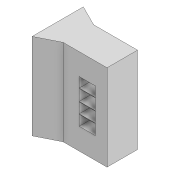
# Autodesk Inventor part: Sliding test insert
Saved by Autodesk Inventor 2020 (Build 240168000, 168)
## iProperties
Created: 2019-11-10
Part Number: Sliding test insert
Material: Generic
Document SubType Name: Modeling
Designer: ball
Density: 1 g/cm^3
Appearance: Default
Author: ball
Autodesk Inventor part; units mm, degrees
ref_plane "YZ Plane" through (0, 0, 0) normal (1, 0, 0) x (0, 1, 0)
ref_plane "XZ Plane" through (0, 0, 0) normal (0, 1, 0) x (-1, 0, 0)
ref_plane "XY Plane" through (0, 0, 0) normal (0, 0, 1) x (1, 0, 0)
sketch "Sketch1" plane through (0, 0, 0) normal (0, 1, 0) x (-1, 0, 0)
  line L0 (0, 4.5) -> (-12.7, 4.5)
  line L1 (-12.7, 4.5) -> (-12.7, -4.5)
  line L2 (-12.7, -4.5) -> (0, -4.5)
  line L3 (0, 4.5) -> (0.254, 4.5)
  line L4 (0.254, -4.5) -> (0, -4.5)
  line L5 (6.35, 4.5) -> (6.35, -4.5)
  line L6 (6.35, 7.548) -> (6.35, 4.5)
  line L7 (6.35, -7.548) -> (6.35, -4.5)
  line L8 (0.254, 4.5) -> (6.35, 7.548)
  line L9 (0.254, -4.5) -> (6.35, -7.548)
  point P0 (0, 0)
  point P1 (0, -4.5)
  dimension "d1" = 9
  dimension "d2" = 4.5
  dimension "d7" = 3.048
  dimension "d8" = 3.048
  dimension "d9" = 12.954
  dimension "d16" = 6.096
  constraints: 20 end point, 2 horizontal, 2 parallel, 2 point on line, 1 perpendicular
  measures "d1" distance of L1.end L0.end
  measures "d2" distance from line of L0 point (0, 0)
  measures "d7" distance from line of L6.start L0
  measures "d8" distance from line of L7.start L2
  measures "d9" distance from line of L4.start L1
  measures "d16" distance from line of L7 L4.start
extrude "Shape" add sketch "Sketch1" along normal blind 25.4
sketch "Sketch2" plane through (-0.254, 0, 4.5) normal (0, 0, 1) x (1, 0, 0)
  line L0 (4.7625, 19.05) -> (9.5125, 19.05)
  line L1 (9.5125, 19.05) -> (9.5125, 6.35)
  line L2 (9.5125, 6.35) -> (4.7625, 6.35)
  line L3 (4.7625, 6.35) -> (4.7625, 19.05)
  point P0 (0.254, 0)
  dimension "d12" = 4.75
  dimension "d13" = 12.7
  constraints: 8 end point, 2 parallel, 1 horizontal, 1 perpendicular
  measures "d12" distance of L1.end L2.end
  measures "d13" distance of L0.end L1.end
extrude "Bridge" cut sketch "Sketch2" against normal through all
sketch "Sketch3" plane through (4.5085, 6.35, 4.5) normal (1, 0, 0) x (0, 0, -1)
  line L0 (9, 12.7) -> (9, 0) construction
  line L1 (0, 12.7) -> (9, 12.7) construction
  line L2 (9, 0) -> (0, 0) construction
  line L3 (0, -6.35) -> (0, 19.05) projected
  line L4 (9, -6.35) -> (9, 19.05) projected
  line L5 (0, 9.7549) -> (9, 9.7549)
  line L6 (9, 9.7549) -> (9, 9.6279)
  line L7 (9, 9.6279) -> (0, 9.6279)
  line L8 (0, 9.6279) -> (0, 9.7549)
  line L9 (0, 6.35) -> (9, 6.35)
  line L10 (9, 6.35) -> (9, 6.223)
  line L11 (9, 6.223) -> (0, 6.223)
  line L12 (0, 6.223) -> (0, 6.35)
  line L13 (0, 3.175) -> (9, 3.175)
  line L14 (9, 3.175) -> (9, 3.048)
  line L15 (9, 3.048) -> (0, 3.048)
  line L16 (0, 3.048) -> (0, 3.175)
  point P0 (4.5, -6.35)
  point P1 (0, 3.048)
  point P2 (0, 6.223)
  point P3 (9, 6.35)
  point P4 (0, 9.6279)
  point P5 (9, 9.7549)
  dimension "d17" = 0.127
  dimension "d18" = 0.127
  dimension "d19" = 0.127
  dimension "d20" = 2.9451
  dimension "d22" = 9.525
  constraints: 28 end point, 6 parallel, 5 horizontal, 4 point on line, 3 perpendicular, 1 midpoint
  measures "d17" distance of L5.end L6.end
  measures "d18" distance of L9.end L10.end
  measures "d19" distance of L13.end L14.end
  measures "d20" distance between parallel lines of L1 L5
  measures "d22" distance between parallel lines of L13 L1
extrude "Supports" add sketch "Sketch3" along normal up to surface (4.75 mm away) contours L3 L13 L4 L15 | L3 L9 L4 L11 | L3 L5 L4 L7
equation "\"d8\" = d7"
equation "\"d18\" = d17"
equation "\"d19\" = d17"
body "Solid1"
